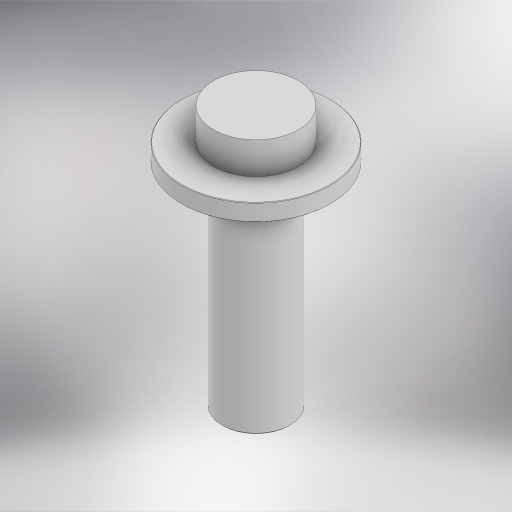
# Autodesk Inventor part: Stempel
Saved by Autodesk Inventor 2023 (Build 270158000, 158)
## iProperties
Created: 2022-11-23
Part Number: Stempel
Material: Generisch
Document SubType Name: Modeling
Designer: schil
Density: 1 g/cm^3
Appearance: Vorgabe
Author: schil
Autodesk Inventor part; units mm, degrees
ref_plane "YZ Plane" through (0, 0, 0) normal (1, 0, 0) x (0, 1, 0)
ref_plane "XZ Plane" through (0, 0, 0) normal (0, 1, 0) x (-1, 0, 0)
ref_plane "XY Plane" through (0, 0, 0) normal (0, 0, 1) x (1, 0, 0)
sketch "Skizze1" plane through (0, 0, 0) normal (1, 0, 0) x (0, 1, 0)
  line L0 (8, 0) -> (0, 0)
  line L1 (0, 0) -> (0, -35)
  line L2 (0, -35) -> (8, -35)
  line L3 (8, -35) -> (8, 0)
  line L4 (23, 0) -> (8, 0)
  line L5 (8, 0) -> (8, -20)
  line L6 (8, -20) -> (23, -20)
  line L7 (23, -20) -> (23, 0)
  dimension "d0" = 20
  dimension "d1" = 35
  dimension "d2" = 8
  dimension "d3" = 15
  constraints: 16 end point, 4 parallel, 2 horizontal, 2 perpendicular, 2 point on line, 1 coincident
  measures "d0" distance of L6.end L4.start
  measures "d1" distance of L0.end L1.end
  measures "d2" distance of L1.end L2.end
  measures "d3" distance of L5.end L6.end
revolve "Umdrehung1" add sketch "Skizze1" angle 360 about axis through (0, 23, 0) along (0, -1, 0)
chamfer "Fase1" distance 0.25 angle 45 2 edges at (0, 8, 35) (0, 0, 35)
sketch "Skizze2" plane through (0, 0, 0) normal (0, -1, 0) x (1, 0, 0)
  circle A0 centre (0, 0) radius 16
  dimension "d8" = 32
  constraints: 1 centre point, 1 coincident
  measures "d8" diameter of A0
extrude "Extrusion1" add sketch "Skizze2" along normal blind 100
chamfer "Fase2" distance 0.5 angle 45 1 edges at (-16, -100, 0)
